Autodesk Fusion 360 part; units mm, degrees
(part 5 of 5)
equation "addendum = ( 1 / diametricalpitch * 1 mm ) * 10 mm"
equation "dedendum = ( 2 / diametricalpitch * 1 mm ) * 10 mm"
equation "rackteeth = 17"
equation "racktoothpitch = ( 1.75 * PI / diametricalpitch * 1 mm ) * 10 mm"
equation "outercirclediam = ( 0.5 * ( PI * cos(pressureangle) / diametricalpitch ) * 1 mm ) * 10 mm"
equation "d72 = ( 360 / 16 / 2 ) * 1 deg"
equation "d78 = addendum"
equation "d79 = dedendum"
equation "d82 = backlash"
equation "d85 = thickness"
equation "d87 = rackteeth"
equation "d89 = racktoothpitch"
equation "d90 = racktoothpitch"
equation "d144 = ( 8 / 2 ) * 1 mm"
equation "d155 = ( 8 / 2 ) * 1 mm"
named bodies: "Base", "Arm", "Handle"
